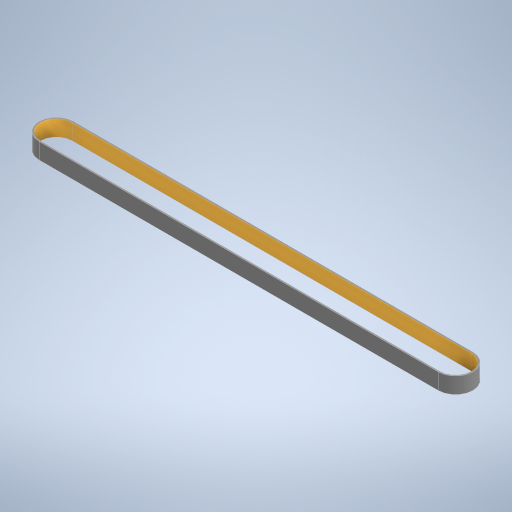
# Autodesk Inventor part: belt
Saved by Autodesk Inventor 2024.1 (Build 281209000, 209)
## iProperties
Created: 2025-03-04
Part Number: belt
Material: 一般
Document SubType Name: Modeling
Designer: hibik
Density: 1 g/cm^3
Appearance: 既定
Author: hibik
Autodesk Inventor part; units mm, degrees
ref_plane "YZ Plane" through (0, 0, 0) normal (1, 0, 0) x (0, 1, 0)
ref_plane "XZ Plane" through (0, 0, 0) normal (0, 1, 0) x (-1, 0, 0)
ref_plane "XY Plane" through (0, 0, 0) normal (0, 0, 1) x (1, 0, 0)
sketch "スケッチ1" plane through (0, 0, 0) normal (0, 1, 0) x (-1, 0, 0)
  line L0 (75, 6.5) -> (-75, 6.5)
  line L1 (-75, -6.5) -> (75, -6.5)
  line L2 (0, -9.1) -> (0, 9.1) projected
  line L3 (75, 6.5) -> (75, -6.5) construction
  line L4 (-75, 6.5) -> (-75, -6.5) construction
  circle A0 centre (75, 0) radius 6.5
  circle A1 centre (-75, 0) radius 6.5
  circle A2 centre (75, 0) radius 6
  circle A3 centre (-75, 0) radius 6
  line L5 (75, -6) -> (-75, -6)
  line L6 (-75, 6) -> (75, 6)
  point P0 (0, 0)
  point P1 (75, 6.5)
  point P2 (-75, 6.5)
  dimension "d3" = 13
  dimension "d2" = 150
  dimension "d4" = 12
  dimension "d5" = 12
  constraints: 12 end point, 4 point on circle, 4 point on line, 3 coincident, 2 centre point, 2 midpoint, 2 vertical, 1 horizontal, 1 horizontal alignment, 1 parallel, 7 other
  measures "d2" distance of L0.start L0.end
  measures "d4" diameter of A2
  measures "d5" diameter of A3
extrude "押し出し1" add sketch "スケッチ1" along normal blind 6 contours A0 L6 L2 L0 | A0 L5 A2 L6 | L2 L6 A1 L0 | A1 L6 A3 L5 | L1 L2 L5 A0 | A1 L5 L2 L1 picked at (80.8664, -2.29) picked at (-77.4549, -5.7931)
